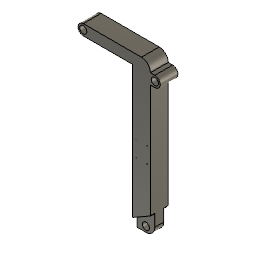
upper_leg (Autodesk Fusion 360 design; units mm, degrees)
part number: 2025-10-29-16-17-56-487
Autodesk Fusion 360 part; units mm, degrees
sketch "Sketch1" plane through (0, 0, 0) normal (0, 1, 0) x (1, 0, 0)
  line L0 (0, 0) -> (12.7, 0)
  line L1 (25.4, -12.7) -> (25.4, -218.44)
  line L2 (25.4, -218.44) -> (0, -218.44)
  line L3 (0, -218.44) -> (0, 0)
  line L4 (0, -218.44) -> (-77.47, -218.44)
  line L5 (-77.47, -218.44) -> (-77.47, -203.2)
  line L6 (-77.47, -203.2) -> (0, -203.2)
  line L7 (0, -203.2) -> (0, -218.44)
  line L8 (25.4, -205.74) -> (39.37, -205.74)
  line L9 (39.37, -205.74) -> (39.37, -190.5)
  line L10 (39.37, -190.5) -> (25.4, -190.5)
  line L11 (25.4, -190.5) -> (25.4, -205.74)
  circle A0 centre (-69.85, -210.82) radius 5.08
  circle A1 centre (31.75, -198.12) radius 5.08
  circle A2 centre (12.7, -7.62) radius 5.08
  arc A3 (25.4, -12.7) -> (12.7, 0) centre (12.7, -12.7) ccw
  point P0 (25.4, 0)
  dimension "d1" = 25.4
  dimension "d2" = 218.44
  dimension "d3" = 77.47
  dimension "d4" = 15.24
  dimension "d5" = 13.97
  dimension "d6" = 15.24
  dimension "d7" = 10.16
  dimension "d8" = 10.16
  dimension "d9" = 10.16
  dimension "d10" = 12.7
  dimension "d11" = 7.62
  dimension "d12" = 190.5
  dimension "d13" = 7.62
  dimension "d14" = 7.62
  dimension "d15" = 7.62
  dimension "d16" = 7.62
  dimension "d17" = 12.7
  constraint horizontal L0
  constraint vertical L1
  constraint horizontal L2
  constraint vertical L3
  constraint coincident L0.start L3.end
  constraint horizontal L4
  constraint vertical L5
  constraint horizontal L6
  constraint vertical L7
  constraint horizontal L8
  constraint vertical L9
  constraint horizontal L10
  constraint vertical L11
  constraint coincident L1 L8.start
  constraint coincident P0 L0
  constraint coincident P0 L1
  constraint tangent L0 A3
  constraint tangent L1 A3
  measures "d1" distance of L0.start P0
  measures "d2" distance of L0.start L2.end
  measures "d3" distance of L2.end L4.end
  measures "d4" distance of L2.end L6.end
  measures "d5" distance of L8.start L8.end
  measures "d6" distance of L8.start L10.end
  measures "d7" diameter of A0
  measures "d8" diameter of A1
  measures "d9" diameter of A2
  measures "d10" distance of L1 A2.centre
  measures "d11" distance of L0 A2.centre
  measures "d12" vertical distance of A1.centre A2.centre
  measures "d13" distance of L9 A1.centre
  measures "d14" distance of L8 A1.centre
  measures "d15" distance of L5 A0.centre
  measures "d16" distance of L4 A0.centre
  measures "d17" radius of A3
extrude "Extrude1" add sketch "Sketch1" along normal blind 25.4
sketch "Sketch2" plane through (0, 0, 0) normal (0, -1, 0) x (1, 0, 0)
  circle A0 centre (-69.85, 210.82) radius 5.08
  circle A1 centre (31.75, 198.12) radius 5.08
  circle A2 centre (12.7, 7.62) radius 5.08
  line L0 (39.37, 205.74) -> (25.4, 205.74)
  line L1 (25.4, 205.74) -> (25.4, 218.44)
  line L2 (25.4, 218.44) -> (-77.47, 218.44)
  line L3 (-77.47, 218.44) -> (-77.47, 203.2)
  line L4 (-77.47, 203.2) -> (0, 203.2)
  line L5 (0, 203.2) -> (0, 0)
  line L6 (0, 0) -> (12.7, 0)
  arc A3 (12.7, 0) -> (25.4, 12.7) centre (12.7, 12.7) ccw
  line L7 (25.4, 12.7) -> (25.4, 190.5)
  line L8 (25.4, 190.5) -> (39.37, 190.5)
  line L9 (39.37, 190.5) -> (39.37, 205.74)
  line L10 (0, 0) -> (0, 20.32)
  line L11 (25.4, 20.32) -> (0, 20.32)
  line L12 (25.4, 20.32) -> (25.4, 12.7)
  line L13 (0, 0) -> (12.7, 0)
  arc A4 (12.7, 0) -> (25.4, 12.7) centre (12.7, 12.7) ccw
  constraint coincident L5.end L6.start
  constraint coincident L5 L10.end
  constraint coincident L7 L11.start
  constraint perpendicular L5 L11
  constraint coincident A3.end L7.start
  constraint coincident L6.end A3.start
  constraint tangent L6 A4
extrude "Extrude2" cut sketch "Sketch2" against normal blind 6.3576 contours L5 L6 A3 L7 L10 L11 L12 L13 A4
sketch "Sketch3" plane through (0, 25.4, 0) normal (0, 1, 0) x (-1, 0, 0)
  circle A0 centre (69.85, 210.82) radius 5.08
  circle A1 centre (-31.75, 198.12) radius 5.08
  circle A2 centre (-12.7, 7.62) radius 5.08
  line L0 (-25.4, 205.74) -> (-39.37, 205.74)
  line L1 (-39.37, 205.74) -> (-39.37, 190.5)
  line L2 (-39.37, 190.5) -> (-25.4, 190.5)
  line L3 (-25.4, 190.5) -> (-25.4, 12.7)
  arc A3 (-25.4, 12.7) -> (-12.7, 0) centre (-12.7, 12.7) ccw
  line L4 (-12.7, 0) -> (0, 0)
  line L5 (0, 0) -> (0, 203.2)
  line L6 (0, 203.2) -> (77.47, 203.2)
  line L7 (77.47, 203.2) -> (77.47, 218.44)
  line L8 (77.47, 218.44) -> (-25.4, 218.44)
  line L9 (-25.4, 218.44) -> (-25.4, 205.74)
  line L10 (0, 0) -> (0, 20.32)
  line L11 (-25.4, 20.32) -> (0, 20.32)
  line L12 (0, 0) -> (-12.7, 0)
  line L13 (-25.4, 20.32) -> (-25.4, 12.7)
  arc A4 (-25.4, 12.7) -> (-12.7, 0) centre (-12.7, 12.7) ccw
  constraint coincident L4.end L5.start
  constraint coincident L5 L10.end
  constraint coincident L3 L11.start
  constraint perpendicular L5 L11
  constraint coincident A3.end L4.start
  constraint coincident L3.end A3.start
  constraint tangent L3 A4
extrude "Extrude3" cut sketch "Sketch3" against normal blind 6.3576 contours L3 A3 L4 L5 L10 L11 L12 L13 A4
extrude "Extrude4" add 1 faces at (16.9333, 2.1192, 20.32) along direction (0, 0, -1) blind 5.5118
sketch "Sketch4" plane through (0, 0, 0) normal (0, -1, 0) x (1, 0, 0)
  line L0 (25.4, 14.8082) -> (25.4, 190.5)
  line L1 (25.4, 190.5) -> (39.37, 190.5)
  line L2 (39.37, 190.5) -> (39.37, 205.74)
  line L3 (39.37, 205.74) -> (25.4, 205.74)
  line L4 (25.4, 205.74) -> (25.4, 218.44)
  line L5 (25.4, 218.44) -> (-77.47, 218.44)
  line L6 (-77.47, 218.44) -> (-77.47, 203.2)
  line L7 (-77.47, 203.2) -> (0, 203.2)
  line L8 (0, 203.2) -> (0, 14.8082)
  line L9 (0, 14.8082) -> (25.4, 14.8082)
  circle A0 centre (-69.85, 210.82) radius 5.08
  circle A1 centre (31.75, 198.12) radius 5.08
  line L10 (0, 14.8082) -> (25.4, 29.4729)
  line L11 (25.4, 29.4729) -> (0, 29.4729)
  line L12 (0, 14.8082) -> (0, 29.4729)
  dimension "d26" = 60
  constraint coincident L8.end L9.start
  constraint coincident L0 L10.end
  constraint coincident L8 L11.end
  constraint perpendicular L8 L11
  measures "d26" angle of L10 L12
extrude "Extrude5" cut sketch "Sketch4" against normal blind 6.3576 contours L0 L9 L10
extrude "Extrude6" add 1 faces at (16.9333, 23.2808, 20.32) along direction (0, 0, -1) blind 5.5118
sketch "Sketch6" plane through (0, 25.4, 0) normal (0, 1, 0) x (-1, 0, 0)
  line L0 (0, 14.8082) -> (0, 203.2)
  line L1 (0, 203.2) -> (77.47, 203.2)
  line L2 (77.47, 203.2) -> (77.47, 218.44)
  line L3 (77.47, 218.44) -> (-25.4, 218.44)
  line L4 (-25.4, 218.44) -> (-25.4, 205.74)
  line L5 (-25.4, 205.74) -> (-39.37, 205.74)
  line L6 (-39.37, 205.74) -> (-39.37, 190.5)
  line L7 (-39.37, 190.5) -> (-25.4, 190.5)
  line L8 (-25.4, 190.5) -> (-25.4, 14.8082)
  line L9 (-25.4, 14.8082) -> (0, 14.8082)
  circle A0 centre (69.85, 210.82) radius 5.08
  circle A1 centre (-31.75, 198.12) radius 5.08
  line L10 (0, 14.8082) -> (-25.4, 29.4729)
  line L11 (-25.4, 29.4729) -> (0, 29.4729)
  line L12 (0, 14.8082) -> (0, 29.4729)
  dimension "d35" = 60
  constraint coincident L0.start L9.end
  constraint coincident L8 L10.end
  constraint coincident L0 L11.end
  constraint perpendicular L0 L11
  measures "d35" angle of L10 L12
extrude "Extrude8" cut sketch "Sketch6" against normal blind 6.3576 contours L8 L9 L10
extrude "Extrude9" cut 2 faces at (16.9333, 4.2384, 24.5847) (16.9333, 21.1616, 24.5847) along direction (-0.5, 0, 0.866025) blind 0.254
fillet "Fillet1" radius 7.62 2 edges at (39.37, 12.7, 205.74) (39.37, 12.7, 190.5)
fillet "Fillet2" radius 7.62 2 edges at (-77.47, 12.7, 218.44) (-77.47, 12.7, 203.2)
fillet "Fillet3" radius 12.7 1 edges at (25.4, 12.7, 218.44)
sketch "Sketch7" plane through (0, 0, 0) normal (0, -1, 0) x (1, 0, 0)
  circle A0 centre (-69.85, 210.82) radius 5.08
  circle A1 centre (31.75, 198.12) radius 5.08
  arc A2 (25.4, 205.74) -> (12.7, 218.44) centre (12.7, 205.74) ccw
  line L0 (12.7, 218.44) -> (-69.85, 218.44)
  arc A3 (-69.85, 218.44) -> (-69.85, 203.2) centre (-69.85, 210.82) ccw
  line L1 (-69.85, 203.2) -> (0, 203.2)
  line L2 (0, 203.2) -> (0, 15.1015)
  line L3 (0, 15.1015) -> (25.273, 29.6929)
  line L4 (25.273, 29.6929) -> (25.4, 29.4729)
  line L5 (25.4, 29.4729) -> (25.4, 190.5)
  line L6 (25.4, 190.5) -> (31.75, 190.5)
  arc A4 (31.75, 190.5) -> (31.75, 205.74) centre (31.75, 198.12) ccw
  line L7 (31.75, 205.74) -> (25.4, 205.74)
  circle A5 centre (5.08, 91.3015) radius 0.3969
  circle A6 centre (20.7518, 91.3015) radius 0.3969
  circle A7 centre (5.08, 113.5265) radius 0.3969
  circle A8 centre (20.7518, 113.5265) radius 0.3969
  dimension "d46" = 0.7937
  dimension "d47" = 0.7937
  dimension "d48" = 0.7937
  dimension "d49" = 0.7937
  dimension "d50" = 15.6718
  dimension "d51" = 15.6718
  dimension "d52" = 22.225
  dimension "d53" = 5.08
  dimension "d54" = 76.2
  measures "d46" diameter of A5
  measures "d47" diameter of A6
  measures "d48" diameter of A7
  measures "d49" diameter of A8
  measures "d50" distance of A5.centre A6.centre
  measures "d51" distance of A7.centre A8.centre
  measures "d52" distance of A5.centre A7.centre
  measures "d53" distance of L2 A5.centre
  measures "d54" vertical distance of L2.end A5.centre
hole "Hole1" at (5.08, 0, 113.5265) at (5.08, 0, 91.3015) at (20.7518, 0, 91.3015) at (20.7518, 0, 113.5265) direction (0, 1, 0) diameter 0.7937 depth 33.02 tip angle 118
